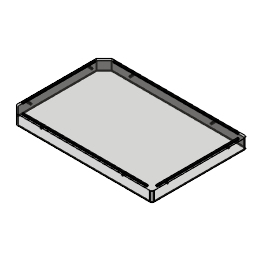
Container V3.0 (Assembly) (Autodesk Fusion 360 archive; units mm, degrees)
design "GREINER 96 WELL PLATE LID"
part number: 2026-02-05-10-27-23-618
Autodesk Fusion 360 part; units mm, degrees
(part 1 of 2)
sketch "Sketch1" plane through (0, 0, 0) normal (0, 0, 1) x (1, 0, 0)
  line L0 (61.42, -42.3) -> (-56.55, -42.3)
  line L1 (-63.55, -35.3) -> (-63.55, 35.3)
  line L2 (-56.55, 42.3) -> (61.42, 42.3)
  line L3 (63.55, 40.17) -> (63.55, -40.17)
  line L4 (63.55, -42.3) -> (-63.55, 42.3) construction
  line L5 (-63.55, -42.3) -> (63.55, 42.3) construction
  line L6 (-56.55, 42.3) -> (-63.55, 35.3)
  line L7 (0, -42.3) -> (0, 42.3) construction
  line L8 (63.55, 0) -> (-63.55, 0) construction
  line L9 (-56.55, -42.3) -> (-63.55, -35.3)
  arc A0 (63.55, 40.17) -> (61.42, 42.3) centre (61.42, 40.17) ccw
  arc A1 (61.42, -42.3) -> (63.55, -40.17) centre (61.42, -40.17) ccw
  dimension "d1" = 84.6
  dimension "d2" = 127.1
  dimension "d3" = 7
  dimension "d4" = 7
  dimension "d5" = 2.13
  constraint horizontal L0
  constraint perpendicular L0 L1
  constraint parallel L0 L2
  constraint parallel L1 L3
  constraint coincident L4 origin
  constraint coincident L5 origin
  constraint coincident L4.end L2
  constraint coincident L4.end L1
  constraint coincident L2 L7.end
  constraint perpendicular L2 L7
  constraint coincident L1 L8.end
  constraint perpendicular L1 L8
  constraint symmetric L2.start L8 L0.end
  constraint symmetric L1.end L8 L1.start
  constraint coincident L0 L7.start
  constraint coincident L3 L8.start
  constraint coincident L5.end L2
  constraint coincident L5.end L3
  constraint tangent L2 A0
  constraint tangent L3 A0
  constraint symmetric L8 L2.end L0.start
  constraint symmetric L8 L3.start L3.end
  constraint symmetric L8 A0 A1
  measures "d1" distance of L5.start L4.end
  measures "d2" distance of L4.end L5.end
  measures "d3" distance of L4.end L2.start
  measures "d4" distance of L4.end L1.end
  measures "d5" radius of A0
extrude "Extrude1" add sketch "Sketch1" against normal blind 9
sketch "Sketch2" plane through (0, 0, -9) normal (0, 0, -1) x (1, 0, 0)
  line L0 (61.42, 42.3) -> (-56.55, 42.3)
  line L1 (-56.55, 42.3) -> (-63.55, 35.3)
  line L2 (-63.55, 35.3) -> (-63.55, -35.3)
  line L3 (-63.55, -35.3) -> (-56.55, -42.3)
  line L4 (-56.55, -42.3) -> (61.42, -42.3)
  arc A0 (61.42, -42.3) -> (63.55, -40.17) centre (61.42, -40.17) ccw
  line L5 (63.55, -40.17) -> (63.55, 40.17)
  arc A1 (63.55, 40.17) -> (61.42, 42.3) centre (61.42, 40.17) ccw
  line L6 (61.42, -41.3) -> (-56.1358, -41.3)
  line L7 (-62.55, -34.8858) -> (-62.55, 34.8858)
  line L8 (-56.1358, 41.3) -> (61.42, 41.3)
  line L9 (62.55, 40.17) -> (62.55, -40.17)
  line L10 (62.55, -41.3) -> (-62.55, 41.3) construction
  line L11 (-62.55, -41.3) -> (62.55, 41.3) construction
  line L12 (-56.1358, 41.3) -> (-62.55, 34.8858)
  arc A2 (62.55, 40.17) -> (61.42, 41.3) centre (61.42, 40.17) ccw
  line L13 (63.55, 0) -> (-63.55, 0) construction
  line L14 (-56.1358, -41.3) -> (-62.55, -34.8858)
  arc A3 (61.42, -41.3) -> (62.55, -40.17) centre (61.42, -40.17) ccw
  dimension "d8" = 125.1
  dimension "d9" = 82.6
  dimension "d10" = 6.4142
  dimension "d11" = 6.4142
  dimension "d12" = 1
  dimension "d13" = 1.13
  constraint horizontal L6
  constraint perpendicular L6 L7
  constraint parallel L6 L8
  constraint parallel L7 L9
  constraint coincident L10 origin
  constraint coincident L11 origin
  constraint coincident L10.end L8
  constraint coincident L10.end L7
  constraint coincident L11.end L9
  constraint coincident L11.end L8
  constraint tangent L9 A2
  constraint tangent L8 A2
  constraint midpoint L5 L13.start
  constraint midpoint L2 L13.end
  constraint symmetric L8.start L13 L6.end
  constraint symmetric L7.end L13 L7.start
  constraint symmetric L9.start L13 L9.end
  constraint symmetric L8.end L13 L6.start
  constraint symmetric A2 L13 A3
  measures "d8" distance of L10.end L11.end
  measures "d9" distance of L11.start L10.end
  measures "d10" distance of L10.end L8.start
  measures "d11" distance of L10.end L7.end
  measures "d12" distance of L1 L12
  measures "d13" radius of A2
extrude "Extrude2" cut sketch "Sketch2" against normal blind 8 contours L6 L7 L8 L9 L12 A2 L14 A3
sketch "Sketch3" plane through (0, 0, -1) normal (0, 0, -1) x (1, 0, 0)
  line L0 (-56.1358, -41.3) -> (61.42, -41.3)
  arc A0 (61.42, -41.3) -> (62.55, -40.17) centre (61.42, -40.17) ccw
  line L1 (62.55, -40.17) -> (62.55, 40.17)
  arc A1 (62.55, 40.17) -> (61.42, 41.3) centre (61.42, 40.17) ccw
  line L2 (61.42, 41.3) -> (-56.1358, 41.3)
  line L3 (-56.1358, 41.3) -> (-62.55, 34.8858)
  line L4 (-62.55, 34.8858) -> (-62.55, -34.8858)
  line L5 (-62.55, -34.8858) -> (-56.1358, -41.3)
  line L6 (-62.55, 32.8642) -> (-35.55, 32.8642) construction
  line L7 (-35.55, 32.8642) -> (-35.55, 41.3) construction
  line L8 (-35.55, 41.3) -> (-36.55, 41.3)
  line L9 (-36.55, 41.3) -> (-36.55, 37.5)
  line L10 (-36.55, 37.5) -> (-35.55, 37.5)
  line L11 (-35.55, 37.5) -> (-35.55, 41.3)
  line L12 (-50.2731, 41.3) -> (-50.2731, 26.6) construction
  line L13 (-50.2731, 26.6) -> (-62.55, 26.6) construction
  line L14 (-62.55, 26.6) -> (-58.75, 26.6)
  line L15 (-58.75, 26.6) -> (-58.75, 27.6)
  line L16 (-58.75, 27.6) -> (-62.55, 27.6)
  line L17 (-62.55, 27.6) -> (-62.55, 26.6)
  line L18 (62.55, 0) -> (-62.55, 0) construction
  line L19 (-62.55, 30.673) -> (-62.55, 55) construction
  line L20 (62.55, 34.8173) -> (62.55, 55) construction
  line L21 (62.55, 55) -> (-62.55, 55) construction
  line L22 (0, 55) -> (0, -41.3) construction
  line L23 (62.55, 27.6) -> (62.55, 26.6)
  line L24 (62.55, 26.6) -> (58.75, 26.6)
  line L25 (58.75, 27.6) -> (62.55, 27.6)
  line L26 (58.75, 26.6) -> (58.75, 27.6)
  line L27 (36.55, 41.3) -> (36.55, 37.5)
  line L28 (35.55, 37.5) -> (35.55, 41.3)
  line L29 (36.55, 37.5) -> (35.55, 37.5)
  line L30 (35.55, 41.3) -> (36.55, 41.3)
  line L31 (62.55, -26.6) -> (58.75, -26.6)
  line L32 (58.75, -27.6) -> (62.55, -27.6)
  line L33 (58.75, -26.6) -> (58.75, -27.6)
  line L34 (35.55, -37.5) -> (35.55, -41.3)
  line L35 (36.55, -37.5) -> (35.55, -37.5)
  line L36 (36.55, -41.3) -> (36.55, -37.5)
  line L37 (62.55, -27.6) -> (62.55, -26.6)
  line L38 (35.55, -41.3) -> (36.55, -41.3)
  line L39 (-58.75, -26.6) -> (-58.75, -27.6)
  line L40 (-62.55, -26.6) -> (-58.75, -26.6)
  line L41 (-58.75, -27.6) -> (-62.55, -27.6)
  line L42 (-62.55, -27.6) -> (-62.55, -26.6)
  line L43 (-36.55, -37.5) -> (-35.55, -37.5)
  line L44 (-35.55, -37.5) -> (-35.55, -41.3)
  line L45 (-36.55, -41.3) -> (-36.55, -37.5)
  line L46 (-35.55, -41.3) -> (-36.55, -41.3)
  dimension "d16" = 27
  dimension "d17" = 3.8
  dimension "d18" = 1
  dimension "d19" = 14.7
  dimension "d20" = 3.8
  dimension "d21" = 1
  constraint coincident L4 L6.start
  constraint perpendicular L4 L6
  constraint coincident L2 L7.end
  constraint perpendicular L2 L7
  constraint horizontal L8
  constraint vertical L9
  constraint horizontal L10
  constraint vertical L11
  constraint coincident L2 L12.start
  constraint perpendicular L2 L12
  constraint coincident L4 L13.end
  constraint perpendicular L4 L13
  constraint horizontal L14
  constraint vertical L15
  constraint horizontal L16
  constraint vertical L17
  constraint midpoint L1 L18.start
  constraint midpoint L4 L18.end
  constraint coincident L4 L19.start
  constraint perpendicular L6 L19
  constraint coincident L1 L20.start
  constraint parallel L1 L20
  constraint perpendicular L19 L21
  constraint midpoint L21 L22.start
  constraint coincident L0 L22.end
  constraint perpendicular L0 L22
  constraint symmetric L7.end L22 L28.end
  constraint symmetric L8.end L22 L27.start
  constraint symmetric L9.end L22 L27.end
  constraint symmetric L10.end L22 L28.start
  constraint symmetric L13.end L22 L23.end
  constraint symmetric L14.end L22 L24.end
  constraint symmetric L15.end L22 L25.start
  constraint symmetric L16.end L22 L23.start
  constraint symmetric L7.end L18 L44.end
  constraint symmetric L8.end L18 L45.start
  constraint symmetric L9.end L18 L43.start
  constraint symmetric L10.end L18 L43.end
  constraint symmetric L13.end L18 L40.start
  constraint symmetric L14.end L18 L39.start
  constraint symmetric L15.end L18 L39.end
  constraint symmetric L16.end L18 L41.end
  constraint symmetric L18 L23.start L32.end
  constraint symmetric L18 L23.end L31.start
  constraint symmetric L18 L27.end L35.start
  constraint symmetric L18 L28.start L34.start
  constraint symmetric L18 L24.end L31.end
  constraint symmetric L18 L25.start L32.start
  constraint symmetric L18 L27.start L36.start
  constraint symmetric L18 L28.end L34.end
  measures "d16" distance of L6.start L6.end
  measures "d17" distance of L8.end L9.end
  measures "d18" distance of L9.end L10.end
  measures "d19" distance of L12.start L12.end
  measures "d20" distance of L15.end L16.end
  measures "d21" distance of L14.end L15.end
extrude "Extrude3" add sketch "Sketch3" along normal blind 1 contours L0 L43 L44 L45 L46 | L4 L39 L40 L41 L42 | L0 L34 L35 L36 L38 | L4 L14 L15 L16 L17 | L1 L31 L32 L33 L37 | L2 L8 L9 L10 L11 | L1 L23 L24 L25 L26 | L2 L27 L28 L29 L30
sketch "Sketch4" plane through (0, 0, 0) normal (0, 0, 1) x (-1, 0, 0)
  line L0 (56.55, 42.3) -> (-61.42, 42.3)
  arc A0 (-61.42, 42.3) -> (-63.55, 40.17) centre (-61.42, 40.17) ccw
  line L1 (-63.55, 40.17) -> (-63.55, -40.17)
  arc A1 (-63.55, -40.17) -> (-61.42, -42.3) centre (-61.42, -40.17) ccw
  line L2 (-61.42, -42.3) -> (56.55, -42.3)
  line L3 (56.55, -42.3) -> (63.55, -35.3)
  line L4 (63.55, -35.3) -> (63.55, 35.3)
  line L5 (63.55, 35.3) -> (56.55, 42.3)
  line L6 (-63.55, -34.3916) -> (-62.25, -34.3916) construction
  line L7 (-62.25, -34.3916) -> (-62.25, -36.4) construction
  line L8 (-60, -42.3) -> (-66.2, -42.3) construction
  line L9 (-63.55, -39.2433) -> (-63.55, -43.1) construction
  line L10 (-62.25, -36.4) -> (-60.95, -36.4)
  line L11 (-60.95, -36.4) -> (-60.95, 36.4)
  line L12 (-60.95, 36.4) -> (-62.25, 36.4)
  line L13 (-62.25, 36.4) -> (-62.25, -36.4)
  line L14 (-52.6219, -42.3) -> (-52.6219, -41) construction
  line L15 (-52.6219, -41) -> (-57.65, -41) construction
  line L16 (-57.65, -41) -> (53.05, -41)
  line L17 (53.05, -41) -> (53.05, -39.7)
  line L18 (53.05, -39.7) -> (-57.65, -39.7)
  line L19 (-57.65, -39.7) -> (-57.65, -41)
  line L20 (53.05, 39.7) -> (-57.65, 39.7)
  line L21 (-57.65, 41) -> (53.05, 41)
  line L22 (-57.65, 39.7) -> (-57.65, 41)
  line L23 (53.05, 41) -> (53.05, 39.7)
  line L24 (60.95, 0) -> (60.95, -32.3)
  line L25 (60.95, -32.3) -> (62.25, -32.3)
  line L26 (62.25, -32.3) -> (62.25, 0)
  line L27 (60.95, 0) -> (60.95, 32.3)
  line L28 (62.25, 32.3) -> (62.25, 0)
  line L29 (60.95, 32.3) -> (62.25, 32.3)
  line L30 (-63.55, 0) -> (60.95, 0) construction
  line L31 (62.25, 0) -> (63.55, 0) construction
  dimension "d24" = 1.3
  dimension "d25" = 5.9
  dimension "d26" = 72.8
  dimension "d27" = 1.3
  dimension "d28" = 1.3
  dimension "d29" = 5.9
  dimension "d30" = 1.3
  dimension "d31" = 110.7
  dimension "d32" = 32.3
  dimension "d33" = 1.3
  dimension "d34" = 1.3
  constraint coincident L1 L6.start
  constraint perpendicular L1 L6
  constraint perpendicular L6 L7
  constraint coincident L2 L8.start
  constraint parallel L2 L8
  constraint coincident L1 L9.start
  constraint perpendicular L2 L9
  constraint horizontal L10
  constraint vertical L11
  constraint horizontal L12
  constraint vertical L13
  constraint coincident L2 L14.start
  constraint perpendicular L2 L14
  constraint perpendicular L14 L15
  constraint horizontal L16
  constraint vertical L17
  constraint horizontal L18
  constraint vertical L19
  constraint midpoint L1 L30.start
  constraint midpoint L4 L31.end
  constraint symmetric L15.end L21.start L30
  constraint symmetric L16.end L21.end L30
  constraint symmetric L17.end L20.start L30
  constraint symmetric L18.end L20.end L30
  constraint vertical L24
  constraint horizontal L25
  constraint vertical L26
  constraint symmetric L24.end L27.end L30
  constraint symmetric L25.end L28.start L31
  constraint collinear L30 L31
  measures "d24" distance of L6.start L6.end
  measures "d25" distance of L7.end L8
  measures "d26" distance of L10.end L11.end
  measures "d27" distance of L7.end L10.end
  measures "d28" distance of L14.start L14.end
  measures "d29" distance of L9 L15.end
  measures "d30" distance of L15.end L18.end
  measures "d31" distance of L17.end L18.end
  measures "d32" distance of L24.start L24.end
  measures "d33" distance of L24.end L25.end
  measures "d34" distance of L4 L26
extrude "Extrude4" add sketch "Sketch4" along normal blind 1 contours L10 L11 L12 L13 | L16 L17 L18 L19 | L20 L21 L22 L23 | L24 L25 L26 L27 L28 L29
equation "d4 = d3"
equation "d11 = d10"

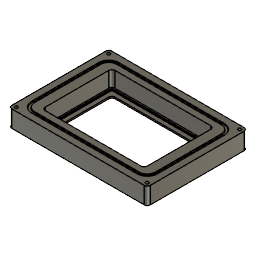
design "Base V3.0"
part number: 2026-01-30-14-30-51-369
Autodesk Fusion 360 part; units mm, degrees
sketch "Sketch1" plane through (0, 0, 0) normal (0, 0, 1) x (1, 0, 0)
  line L0 (86, -65) -> (-86, -65)
  line L1 (-90, -61) -> (-90, 61)
  line L2 (-86, 65) -> (86, 65)
  line L3 (90, 61) -> (90, -61)
  line L4 (90, -65) -> (-90, 65) construction
  line L5 (-90, -65) -> (90, 65) construction
  arc A0 (-86, 65) -> (-90, 61) centre (-86, 61) ccw
  arc A1 (90, 61) -> (86, 65) centre (86, 61) ccw
  arc A2 (86, -65) -> (90, -61) centre (86, -61) ccw
  arc A3 (-90, -61) -> (-86, -65) centre (-86, -61) ccw
  circle A4 centre (-85, 60) radius 2
  line L6 (0, 65) -> (0, -65) construction
  line L7 (90, 0) -> (-90, 0) construction
  circle A5 centre (85, 60) radius 2
  circle A6 centre (85, -60) radius 2
  circle A7 centre (-85, -60) radius 2
  dimension "d1" = 180
  dimension "d2" = 130
  dimension "d26" = 4
  dimension "d27" = 4
  dimension "d28" = 4
  dimension "d29" = 4
  dimension "d30" = 4
  dimension "d31" = 5
  dimension "d32" = 5
  constraint horizontal L0
  constraint perpendicular L0 L1
  constraint parallel L0 L2
  constraint parallel L1 L3
  constraint coincident L4 origin
  constraint coincident L5 origin
  constraint coincident L4.end L2
  constraint coincident L4.end L1
  constraint tangent L2 A0
  constraint tangent L1 A0
  constraint coincident L5.end L3
  constraint coincident L5.end L2
  constraint tangent L3 A1
  constraint tangent L2 A1
  constraint coincident L4.start L3
  constraint coincident L4.start L0
  constraint tangent L3 A2
  constraint tangent L0 A2
  constraint coincident L5.start L1
  constraint coincident L5.start L0
  constraint tangent L1 A3
  constraint tangent L0 A3
  constraint midpoint L2 L6.start
  constraint midpoint L0 L6.end
  constraint midpoint L3 L7.start
  constraint midpoint L1 L7.end
  constraint symmetric A4 L6 A5
  constraint symmetric A4 L7 A7
  constraint symmetric L7 A5 A6
  measures "d1" distance of L4.end L5.end
  measures "d2" distance of L5.start L4.end
  measures "d26" radius of A0
  measures "d27" radius of A1
  measures "d28" radius of A2
  measures "d29" radius of A3
  measures "d30" diameter of A4
  measures "d31" distance of L2 A4.centre
  measures "d32" distance of L1 A4.centre
extrude "Extrude1" add sketch "Sketch1" along normal blind 22
sketch "Sketch2" plane through (0, 0, 22) normal (0, 0, 1) x (-1, 0, 0)
  line L0 (-86, -65) -> (86, -65)
  line L1 (90, -61) -> (90, 61)
  line L2 (86, 65) -> (-86, 65)
  line L3 (-90, 61) -> (-90, -61)
  line L4 (-62.2, 45.25) -> (62.2, 45.25)
  line L5 (66.2, 41.25) -> (66.2, -41.25)
  line L6 (62.2, -45.25) -> (-62.2, -45.25)
  line L7 (-66.2, -41.25) -> (-66.2, 41.25)
  line L8 (-66.2, 45.25) -> (66.2, -45.25) construction
  line L9 (66.2, 45.25) -> (-66.2, -45.25) construction
  arc A0 (86, -65) -> (90, -61) centre (86, -61) ccw
  arc A1 (90, 61) -> (86, 65) centre (86, 61) ccw
  arc A2 (-86, 65) -> (-90, 61) centre (-86, 61) ccw
  arc A3 (-90, -61) -> (-86, -65) centre (-86, -61) ccw
  circle A4 centre (85, 60) radius 2
  circle A5 centre (-85, 60) radius 2
  circle A6 centre (-85, -60) radius 2
  circle A7 centre (85, -60) radius 2
  arc A8 (62.2, -45.25) -> (66.2, -41.25) centre (62.2, -41.25) ccw
  arc A9 (-66.2, -41.25) -> (-62.2, -45.25) centre (-62.2, -41.25) ccw
  arc A10 (66.2, 41.25) -> (62.2, 45.25) centre (62.2, 41.25) ccw
  arc A11 (-62.2, 45.25) -> (-66.2, 41.25) centre (-62.2, 41.25) ccw
  dimension "d5" = 132.4
  dimension "d6" = 90.5
  dimension "d52" = 4
  dimension "d53" = 4
  dimension "d54" = 4
  dimension "d55" = 4
  constraint horizontal L4
  constraint perpendicular L4 L5
  constraint parallel L4 L6
  constraint parallel L5 L7
  constraint coincident L8 origin
  constraint coincident L9 origin
  constraint coincident L8.end L6
  constraint coincident L8.end L5
  constraint tangent L6 A8
  constraint tangent L5 A8
  constraint coincident L9.end L6
  constraint coincident L9.end L7
  constraint tangent L6 A9
  constraint tangent L7 A9
  constraint coincident L9.start L5
  constraint coincident L9.start L4
  constraint tangent L5 A10
  constraint tangent L4 A10
  constraint coincident L8.start L7
  constraint coincident L8.start L4
  constraint tangent L7 A11
  constraint tangent L4 A11
  measures "d5" distance of L8.end L9.end
  measures "d6" distance of L9.start L8.end
  measures "d52" radius of A8
  measures "d53" radius of A9
  measures "d54" radius of A10
  measures "d55" radius of A11
extrude "Extrude2" cut sketch "Sketch2" against normal blind 20 contours L4 L5 L6 L7 A8 A9 A10 A11
sketch "Sketch3" plane through (0, 0, 22) normal (0, 0, 1) x (-1, 0, 0)
  line L0 (66.2, 41.25) -> (66.2, -41.25)
  line L1 (62.2, -45.25) -> (-62.2, -45.25)
  line L2 (-66.2, -41.25) -> (-66.2, 41.25)
  line L3 (-62.2, 45.25) -> (62.2, 45.25)
  line L4 (-86, -65) -> (86, -65)
  line L5 (90, -61) -> (90, 61)
  line L6 (86, 65) -> (-86, 65)
  line L7 (-90, 61) -> (-90, -61)
  line L8 (-79.9494, 54.9494) -> (79.9494, 54.9494) construction
  line L9 (79.9494, 54.9494) -> (79.9494, -54.9494) construction
  line L10 (79.9494, -54.9494) -> (-79.9494, -54.9494) construction
  line L11 (-79.9494, -54.9494) -> (-79.9494, 54.9494) construction
  line L12 (-79.9494, 54.9494) -> (79.9494, -54.9494) construction
  line L13 (79.9494, 54.9494) -> (-79.9494, -54.9494) construction
  line L14 (78.5149, 43.2459) -> (78.5149, -43.2459)
  line L15 (68.2459, -53.5149) -> (-68.2459, -53.5149)
  line L16 (-78.5149, -43.2459) -> (-78.5149, 43.2459)
  line L17 (-69.5341, 47.3937) -> (78.5149, -53.5149) construction
  line L18 (70.6619, 45.6619) -> (-70.6619, -45.6619) construction
  line L19 (-68.2459, 56.3839) -> (68.2459, 56.3839)
  line L20 (81.3839, 43.2459) -> (81.3839, -43.2459)
  line L21 (68.2459, -56.3839) -> (-68.2459, -56.3839)
  line L22 (-81.3839, -43.2459) -> (-81.3839, 43.2459)
  line L23 (-72.429, 50.1798) -> (81.3839, -56.3839) construction
  line L24 (73.5309, 48.5309) -> (-73.5309, -48.5309) construction
  arc A0 (68.2459, -53.5149) -> (78.5149, -43.2459) centre (68.2459, -43.2459) ccw
  arc A1 (68.2459, -56.3839) -> (81.3839, -43.2459) centre (68.2459, -43.2459) ccw
  line L25 (0, -65) -> (0, 65) construction
  line L26 (-90, 0) -> (90, 0) construction
  arc A2 (-78.5149, -43.2459) -> (-68.2459, -53.5149) centre (-68.2459, -43.2459) ccw
  arc A3 (-81.3839, -43.2459) -> (-68.2459, -56.3839) centre (-68.2459, -43.2459) ccw
  arc A4 (-68.2459, 53.5149) -> (-78.5149, 43.2459) centre (-68.2459, 43.2459) ccw
  arc A5 (-68.2459, 56.3839) -> (-81.3839, 43.2459) centre (-68.2459, 43.2459) ccw
  arc A6 (78.5149, 43.2459) -> (68.2459, 53.5149) centre (68.2459, 43.2459) ccw
  arc A7 (81.3839, 43.2459) -> (68.2459, 56.3839) centre (68.2459, 43.2459) ccw
  line L27 (-68.2459, 53.5149) -> (68.2459, 53.5149)
  arc A8 (86, -65) -> (90, -61) centre (86, -61) ccw
  arc A9 (90, 61) -> (86, 65) centre (86, 61) ccw
  arc A10 (-86, 65) -> (-90, 61) centre (-86, 61) ccw
  arc A11 (-90, -61) -> (-86, -65) centre (-86, -61) ccw
  circle A12 centre (85, 60) radius 2
  circle A13 centre (-85, 60) radius 2
  circle A14 centre (-85, -60) radius 2
  circle A15 centre (85, -60) radius 2
  arc A16 (66.2, 41.25) -> (62.2, 45.25) centre (62.2, 41.25) ccw
  arc A17 (62.2, -45.25) -> (66.2, -41.25) centre (62.2, -41.25) ccw
  arc A18 (-66.2, -41.25) -> (-62.2, -45.25) centre (-62.2, -41.25) ccw
  arc A19 (-62.2, 45.25) -> (-66.2, 41.25) centre (-62.2, 41.25) ccw
  dimension "d9" = 159.8988
  dimension "d15" = 109.8988
  dimension "d16" = 1.4345
  dimension "d17" = 1.4345
  dimension "d18" = 1.4345
  dimension "d19" = 1.4345
  dimension "d20" = 10.269
  dimension "d21" = 13.138
  constraint horizontal L8
  constraint perpendicular L8 L9
  constraint parallel L8 L10
  constraint parallel L9 L11
  constraint coincident L12 origin
  constraint coincident L13 origin
  constraint parallel L15 L27
  constraint parallel L14 L16
  constraint coincident L17 origin
  constraint coincident L18 origin
  constraint horizontal L19
  constraint perpendicular L19 L20
  constraint parallel L19 L21
  constraint parallel L20 L22
  constraint coincident L23 origin
  constraint coincident L24 origin
  constraint coincident L17.end L15
  constraint coincident L17.end L14
  constraint tangent L15 A0
  constraint tangent L14 A0
  constraint coincident L23.end L21
  constraint coincident L23.end L20
  constraint tangent L21 A1
  constraint tangent L20 A1
  constraint midpoint L4 L25.start
  constraint midpoint L6 L25.end
  constraint midpoint L7 L26.start
  constraint midpoint L5 L26.end
  constraint symmetric L15.start L25 L15.end
  constraint symmetric L14.end L25 L16.start
  constraint symmetric A0 L25 A2
  constraint symmetric L21.start L25 L21.end
  constraint symmetric L20.end L25 L22.start
  constraint symmetric A1 L25 A3
  constraint symmetric L15.start L26 A6.end
  constraint symmetric L14.end L26 L14.start
  constraint symmetric A0 L26 A6
  constraint symmetric L21.start L26 L19.end
  constraint symmetric L20.end L26 L20.start
  constraint symmetric A1 L26 A7
  constraint symmetric L26 L15.end A4.start
  constraint symmetric L26 L16.start L16.end
  constraint symmetric L26 A2 A4
  constraint symmetric L26 L21.end L19.start
  constraint symmetric L26 L22.start L22.end
  constraint symmetric L26 A3 A5
  measures "d9" distance of L8.start L8.end
  measures "d15" distance of L8 L10
  measures "d16" distance of L11 L16
  measures "d17" distance of L10 L15
  measures "d18" distance of L11 L22
  measures "d19" distance of L10 L21
  measures "d20" radius of A0
  measures "d21" radius of A1
extrude "Extrude3" cut sketch "Sketch3" against normal blind 1.424 contours L19 L20 L21 L22 A1 A3 A5 A7
draft "Draft1" angle 10 neutral plane through (0, 0, 20.576) pull (0, 0, 1) 16 faces at (-78.5149, -14.4153, 21.5253) (-70.6669, 53.2254, 21.0507) (-22.7486, 53.5149, 21.5253) (74.2025, 51.6108, 21.0507) (78.5149, 14.4153, 21.0507) (71.6046, -52.9501, 21.5253) (22.7486, -53.5149, 21.5253) (-70.6669, -53.2254, 21.0507) (-81.3839, -14.4153, 21.5253) (-68.871, -56.369, 21.0507) (22.7486, -56.3839, 21.0507) (77.7543, -52.3122, 21.0507) (81.3839, 14.4153, 21.5253) (77.3122, 52.7543, 21.0507) (-22.7486, 56.3839, 21.0507) (-73.1288, 55.4428, 21.0507)
sketch "Sketch4" plane through (0, 0, 2) normal (0, 0, 1) x (-1, 0, 0)
  line L0 (-62.2, -45.25) -> (62.2, -45.25)
  line L1 (66.2, -41.25) -> (66.2, 41.25)
  line L2 (62.2, 45.25) -> (-62.2, 45.25)
  line L3 (-66.2, 41.25) -> (-66.2, -41.25)
  line L4 (-52.2, 35.25) -> (52.2, 35.25)
  line L5 (56.2, 31.25) -> (56.2, -31.25)
  line L6 (52.2, -35.25) -> (-52.2, -35.25)
  line L7 (-56.2, -31.25) -> (-56.2, 31.25)
  line L8 (-56.2, 35.25) -> (56.2, -35.25) construction
  line L9 (56.2, 35.25) -> (-56.2, -35.25) construction
  arc A0 (66.2, 41.25) -> (62.2, 45.25) centre (62.2, 41.25) ccw
  arc A1 (-62.2, 45.25) -> (-66.2, 41.25) centre (-62.2, 41.25) ccw
  arc A2 (-66.2, -41.25) -> (-62.2, -45.25) centre (-62.2, -41.25) ccw
  arc A3 (62.2, -45.25) -> (66.2, -41.25) centre (62.2, -41.25) ccw
  arc A4 (52.2, -35.25) -> (56.2, -31.25) centre (52.2, -31.25) ccw
  arc A5 (-56.2, -31.25) -> (-52.2, -35.25) centre (-52.2, -31.25) ccw
  arc A6 (-52.2, 35.25) -> (-56.2, 31.25) centre (-52.2, 31.25) ccw
  arc A7 (56.2, 31.25) -> (52.2, 35.25) centre (52.2, 31.25) ccw
  dimension "d35" = 10
  dimension "d36" = 10
  dimension "d71" = 4
  dimension "d72" = 4
  dimension "d73" = 4
  dimension "d74" = 4
  constraint horizontal L4
  constraint perpendicular L4 L5
  constraint parallel L4 L6
  constraint parallel L5 L7
  constraint coincident L8 origin
  constraint coincident L9 origin
  constraint coincident L8.end L6
  constraint coincident L8.end L5
  constraint tangent L6 A4
  constraint tangent L5 A4
  constraint coincident L9.end L6
  constraint coincident L9.end L7
  constraint tangent L6 A5
  constraint tangent L7 A5
  constraint coincident L8.start L7
  constraint coincident L8.start L4
  constraint tangent L7 A6
  constraint tangent L4 A6
  constraint coincident L9.start L4
  constraint coincident L9.start L5
  constraint tangent L4 A7
  constraint tangent L5 A7
  measures "d35" distance of L3 L7
  measures "d36" distance of L0 L6
  measures "d71" radius of A4
  measures "d72" radius of A5
  measures "d73" radius of A6
  measures "d74" radius of A7
extrude "Extrude4" cut sketch "Sketch4" against normal blind 5 contours L4 L5 L6 L7 A4 A5 A6 A7
sketch "Sketch6" plane through (0, 0, 2) normal (0, 0, 1) x (-1, 0, 0)
  line L0 (56.2, 31.25) -> (56.2, -31.25)
  line L1 (52.2, -35.25) -> (-52.2, -35.25)
  line L2 (-56.2, -31.25) -> (-56.2, 31.25)
  line L3 (-52.2, 35.25) -> (52.2, 35.25)
  arc A0 (66.2, 41.25) -> (62.2, 45.25) centre (62.2, 41.25) ccw
  line L4 (62.2, 45.25) -> (-62.2, 45.25)
  arc A1 (-62.2, 45.25) -> (-66.2, 41.25) centre (-62.2, 41.25) ccw
  line L5 (-66.2, 41.25) -> (-66.2, -41.25)
  arc A2 (-66.2, -41.25) -> (-62.2, -45.25) centre (-62.2, -41.25) ccw
  line L6 (-62.2, -45.25) -> (62.2, -45.25)
  arc A3 (62.2, -45.25) -> (66.2, -41.25) centre (62.2, -41.25) ccw
  line L7 (66.2, -41.25) -> (66.2, 41.25)
  arc A4 (60.9079, -41.3399) -> (62.4799, -39.7679) centre (60.9079, -39.7679) ccw construction
  arc A5 (-62.4799, -39.7399) -> (-60.9079, -41.3119) centre (-60.9079, -39.7399) ccw construction
  line L8 (-48.9575, -41.8399) -> (48.9575, -41.8399) construction
  line L9 (48.9575, 41.8399) -> (-48.9575, 41.8399) construction
  line L10 (-62.9799, 29.7119) -> (-62.9799, 27.8175) construction
  line L11 (48.9575, -41.8399) -> (50.8519, -41.8399) construction
  line L12 (62.4799, 30.3078) -> (62.4799, 39.7679) construction
  arc A6 (-60.88, 42.74) -> (-63.88, 39.74) centre (-60.88, 39.74) ccw construction
  line L13 (63.88, 39.74) -> (63.88, -39.74) construction
  arc A7 (63.88, 39.74) -> (60.88, 42.74) centre (60.88, 39.74) ccw construction
  line L14 (-62.9799, -29.7119) -> (-62.4799, -30.3078) construction
  line L15 (51.4478, 41.3399) -> (50.8519, 41.8399) construction
  arc A8 (60.88, -42.74) -> (63.88, -39.74) centre (60.88, -39.74) ccw construction
  line L16 (-48.9575, 41.8399) -> (-50.8519, 41.8399) construction
  line L17 (-60.88, 42.74) -> (60.88, 42.74) construction
  line L18 (-62.9799, -27.8175) -> (-62.9799, -29.7119) construction
  line L19 (60.88, -42.74) -> (-60.88, -42.74) construction
  line L20 (62.9799, 29.7119) -> (62.4799, 30.3078) construction
  line L21 (-50.8519, 41.8399) -> (-51.4811, 41.3119) construction
  line L22 (62.4799, -39.7679) -> (62.4799, -30.3078) construction
  line L23 (-50.8519, -41.8399) -> (-48.9575, -41.8399) construction
  line L24 (60.9079, 41.3399) -> (51.4478, 41.3399) construction
  line L25 (50.8519, 41.8399) -> (48.9575, 41.8399) construction
  line L26 (62.9799, 27.8175) -> (62.9799, 29.7119) construction
  line L27 (51.4478, -41.3399) -> (60.9079, -41.3399) construction
  line L28 (62.9799, -27.8175) -> (62.9799, 27.8175) construction
  line L29 (-63.88, -39.74) -> (-63.88, 39.74) construction
  line L30 (50.8519, -41.8399) -> (51.4478, -41.3399) construction
  line L31 (62.9799, -29.7119) -> (62.9799, -27.8175) construction
  arc A9 (-63.88, -39.74) -> (-60.88, -42.74) centre (-60.88, -39.74) ccw construction
  arc A10 (62.4799, 39.7679) -> (60.9079, 41.3399) centre (60.9079, 39.7679) ccw construction
  line L32 (62.4799, -30.3078) -> (62.9799, -29.7119) construction
  line L33 (-62.4799, 30.3078) -> (-62.9799, 29.7119) construction
  line L34 (-60.9079, -41.3119) -> (-51.4811, -41.3119) construction
  arc A11 (-60.9079, 41.3119) -> (-62.4799, 39.7399) centre (-60.9079, 39.7399) ccw construction
  line L35 (-51.4811, -41.3119) -> (-50.8519, -41.8399) construction
  line L36 (-51.4811, 41.3119) -> (-60.9079, 41.3119) construction
  line L37 (-62.4799, 39.7399) -> (-62.4799, 30.3078) construction
  line L38 (-62.4799, -30.3078) -> (-62.4799, -39.7399) construction
  line L39 (-62.9799, 27.8175) -> (-62.9799, -27.8175) construction
  line L40 (0, -45.25) -> (0, 45.25) construction
  line L41 (-66.2, 0) -> (66.2, 0) construction
  line L42 (-60.85, 43.25) -> (60.85, 43.25)
  line L43 (64.35, 39.75) -> (64.35, -39.75)
  line L44 (60.85, -43.25) -> (-60.85, -43.25)
  line L45 (-64.35, -39.75) -> (-64.35, 39.75)
  line L46 (-64.35, 43.25) -> (64.35, -43.25) construction
  line L47 (64.35, 43.25) -> (-64.35, -43.25) construction
  arc A12 (60.85, -43.25) -> (64.35, -39.75) centre (60.85, -39.75) ccw
  arc A13 (-64.35, -39.75) -> (-60.85, -43.25) centre (-60.85, -39.75) ccw
  arc A14 (-60.85, 43.25) -> (-64.35, 39.75) centre (-60.85, 39.75) ccw
  arc A15 (64.35, 39.75) -> (60.85, 43.25) centre (60.85, 39.75) ccw
  line L48 (-60.85, 40.75) -> (60.85, 40.75)
  line L49 (61.85, 39.75) -> (61.85, -39.75)
  line L50 (60.85, -40.75) -> (-60.85, -40.75)
  line L51 (-61.85, -39.75) -> (-61.85, 39.75)
  line L52 (-61.85, 40.75) -> (61.85, -40.75) construction
  line L53 (61.85, 40.75) -> (-61.85, -40.75) construction
  arc A16 (-61.85, -39.75) -> (-60.85, -40.75) centre (-60.85, -39.75) ccw
  arc A17 (60.85, -40.75) -> (61.85, -39.75) centre (60.85, -39.75) ccw
  arc A18 (61.85, 39.75) -> (60.85, 40.75) centre (60.85, 39.75) ccw
  arc A19 (-60.85, 40.75) -> (-61.85, 39.75) centre (-60.85, 39.75) ccw
  arc A20 (52.2, -35.25) -> (56.2, -31.25) centre (52.2, -31.25) ccw
  arc A21 (-56.2, -31.25) -> (-52.2, -35.25) centre (-52.2, -31.25) ccw
  arc A22 (-52.2, 35.25) -> (-56.2, 31.25) centre (-52.2, 31.25) ccw
  arc A23 (56.2, 31.25) -> (52.2, 35.25) centre (52.2, 31.25) ccw
  dimension "d56" = 128.7
  dimension "d57" = 86.5
  dimension "d58" = 3.5
  dimension "d59" = 3.5
  dimension "d60" = 3.5
  dimension "d61" = 3.5
  dimension "d63" = 2.5
  dimension "d64" = 2.5
  dimension "d65" = 1
  dimension "d66" = 1
  dimension "d67" = 1
  dimension "d68" = 1
  constraint midpoint L6 L40.start
  constraint midpoint L4 L40.end
  constraint midpoint L5 L41.start
  constraint midpoint L7 L41.end
  constraint horizontal L42
  constraint perpendicular L42 L43
  constraint parallel L42 L44
  constraint parallel L43 L45
  constraint coincident L46 origin
  constraint coincident L47 origin
  constraint coincident L46.end L44
  constraint coincident L46.end L43
  constraint tangent L44 A12
  constraint tangent L43 A12
  constraint coincident L47.end L45
  constraint coincident L47.end L44
  constraint tangent L45 A13
  constraint tangent L44 A13
  constraint coincident L46.start L45
  constraint coincident L46.start L42
  constraint tangent L45 A14
  constraint tangent L42 A14
  constraint coincident L47.start L42
  constraint coincident L47.start L43
  constraint tangent L42 A15
  constraint tangent L43 A15
  constraint horizontal L48
  constraint perpendicular L48 L49
  constraint parallel L48 L50
  constraint parallel L49 L51
  constraint coincident L52 origin
  constraint coincident L53 origin
  constraint coincident L53.end L51
  constraint coincident L53.end L50
  constraint tangent L51 A16
  constraint tangent L50 A16
  constraint coincident L52.end L50
  constraint coincident L52.end L49
  constraint tangent L50 A17
  constraint tangent L49 A17
  constraint coincident L53.start L48
  constraint coincident L53.start L49
  constraint tangent L48 A18
  constraint tangent L49 A18
  constraint coincident L52.start L51
  constraint coincident L52.start L48
  constraint tangent L51 A19
  constraint tangent L48 A19
  measures "d56" distance of L46.end L47.end
  measures "d57" distance of L47.start L46.end
  measures "d58" radius of A12
  measures "d59" radius of A13
  measures "d60" radius of A14
  measures "d61" radius of A15
  measures "d63" distance of L45 L51
  measures "d64" distance of L44 L50
  measures "d65" radius of A16
  measures "d66" radius of A17
  measures "d67" radius of A18
  measures "d68" radius of A19
extrude "Extrude6" cut sketch "Sketch6" against normal blind 1 contours L42 L43 L44 L45 A12 A13 A14 A15
equation "d9 = ( ORingPerimeter - 100 mm ) / 4 + 50 mm"
equation "ORingDiameter = 1.78 mm" comment "Diamter of the O ring"
equation "ORingInnerDiameter = 170 mm" comment "Inner diamter of the o ring bore"
equation "ORingPerimeter = 2 * 3.1412 * ( ( ORingInnerDiameter / 2 ) + ORingDiameter / 2 )"
equation "PanelWidth = 80 mm"
equation "PanelLength = 115 mm"
equation "d15 = ( ORingPerimeter - 100 mm ) / 4"
equation "d16 = ( ( ORingDiameter * 1.05 ) / 2 ) + 0.5 mm"
equation "d17 = ( ( ORingDiameter * 1.05 ) / 2 ) + 0.5 mm"
equation "d18 = ( ( ORingDiameter * 1.05 ) / 2 ) + 0.5 mm"
equation "d19 = ( ( ORingDiameter * 1.05 ) / 2 ) + 0.5 mm"
equation "d20 = ( ORingDiameter ) * 6 + ORingDiameter * 0.05 - 0.5 mm"
equation "d21 = ( ORingDiameter ) * 6 + ( ORingDiameter * 1.1 ) + 0.5 mm"
equation "d22 = -ORingDiameter * 0.8"
equation "ORing2Diameter = 2 mm" comment "Second O ring Diameter"
equation "ORing2InnerDiameter = 126 mm" comment "Inner diameter of the second O Ring"
equation "ORing2Perimeter = 2 * 3.1412 * ( ( ORing2InnerDiameter / 2 ) + ORing2Diameter / 2 )"

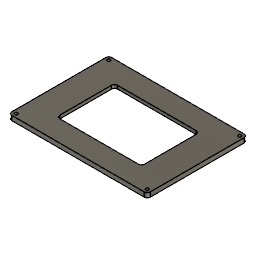
design "Lid V3.0"
part number: 2026-01-29-14-58-12-979
Autodesk Fusion 360 part; units mm, degrees
sketch "Sketch2" plane through (0, 0, 0) normal (0, 0, 1) x (1, 0, 0)
  line L0 (-46, 50) -> (126, 50)
  line L1 (130, 46) -> (130, -76)
  line L2 (126, -80) -> (-46, -80)
  line L3 (-50, -76) -> (-50, 46)
  circle A0 centre (-45, 45) radius 2
  line L4 (40, -80) -> (40, 50) construction
  line L5 (-50, -15) -> (130, -15) construction
  arc A1 (-46, 50) -> (-50, 46) centre (-46, 46) ccw
  circle A2 centre (125, 45) radius 2
  arc A3 (130, 46) -> (126, 50) centre (126, 46) ccw
  circle A4 centre (125, -75) radius 2
  arc A5 (126, -80) -> (130, -76) centre (126, -76) ccw
  circle A6 centre (-45, -75) radius 2
  arc A7 (-50, -76) -> (-46, -80) centre (-46, -76) ccw
  point P0 (-50, 50)
  point P1 (130, 50)
  dimension "d3" = 4
  dimension "d4" = 5
  dimension "d5" = 5
  dimension "d6" = 4
  dimension "d63" = 180
  dimension "d64" = 130
  constraint horizontal L0
  constraint vertical L1
  constraint horizontal L2
  constraint vertical L3
  constraint coincident L0 L4.end
  constraint coincident L3 L5.start
  constraint coincident P0 L0
  constraint coincident P0 L3
  constraint tangent L0 A1
  constraint tangent L3 A1
  constraint symmetric P0 L4 P1
  constraint symmetric A0 L4 A2
  constraint symmetric L4 L0.start L0.end
  constraint symmetric L4 L3.end L1.start
  constraint symmetric L4 A1 A3
  constraint coincident L1 L5.end
  constraint symmetric A0 L5 A6
  constraint symmetric L5 L0.start L2.end
  constraint symmetric L5 L3.end L3.start
  constraint symmetric L5 A1 A7
  constraint symmetric L5 L1.start L1.end
  constraint symmetric L5 L0.end L2.start
  constraint symmetric L5 A2 A4
  constraint symmetric L5 A3 A5
  constraint coincident L2 L4.start
  measures "d3" diameter of A0
  measures "d4" distance of L0 A0.centre
  measures "d5" distance of L3 A0.centre
  measures "d6" radius of A1
  measures "d63" distance of L1 L3
  measures "d64" distance of L0 L2
extrude "Extrude1" add sketch "Sketch2" along normal blind 6
sketch "Sketch3" plane through (0, 0, 0) normal (0, 0, -1) x (1, 0, 0)
  circle A0 centre (125, 75) radius 2
  circle A1 centre (-45, 75) radius 2
  circle A2 centre (-45, -45) radius 2
  circle A3 centre (125, -45) radius 2
  arc A4 (-50, -46) -> (-46, -50) centre (-46, -46) ccw
  line L0 (-46, -50) -> (126, -50)
  arc A5 (126, -50) -> (130, -46) centre (126, -46) ccw
  line L1 (130, -46) -> (130, 76)
  arc A6 (130, 76) -> (126, 80) centre (126, 76) ccw
  line L2 (126, 80) -> (-46, 80)
  arc A7 (-46, 80) -> (-50, 76) centre (-46, 76) ccw
  line L3 (-50, 76) -> (-50, -46)
  line L4 (40, 80) -> (40, -50) construction
  line L5 (130, 15) -> (-50, 15) construction
  line L6 (119.9494, -39.9494) -> (-39.9494, -39.9494) construction
  line L7 (-39.9494, -39.9494) -> (-39.9494, 69.9494) construction
  line L8 (-39.9494, 69.9494) -> (119.9494, 69.9494) construction
  line L9 (119.9494, 69.9494) -> (119.9494, -39.9494) construction
  line L10 (119.9494, -39.9494) -> (-39.9494, 69.9494) construction
  line L11 (-39.9494, -39.9494) -> (119.9494, 69.9494) construction
  line L12 (108.2459, -41.3839) -> (-28.2459, -41.3839)
  line L13 (-41.3839, -28.2459) -> (-41.3839, 58.2459)
  line L14 (-28.2459, 71.3839) -> (108.2459, 71.3839)
  line L15 (121.3839, 58.2459) -> (121.3839, -28.2459)
  line L16 (95.6336, -23.5438) -> (-41.3839, 71.3839) construction
  line L17 (-38.6963, -33.1786) -> (83.6146, 41.7012) construction
  line L18 (-38.5149, -28.2459) -> (-38.5149, 58.2459)
  line L19 (-28.2459, 68.5149) -> (108.2459, 68.5149)
  line L20 (118.5149, 58.2459) -> (118.5149, -28.2459)
  line L21 (104.513, -28.9713) -> (-38.5149, 68.5149) construction
  line L22 (-36.0332, -30.305) -> (80.8211, 39.3236) construction
  arc A8 (-28.2459, 68.5149) -> (-38.5149, 58.2459) centre (-28.2459, 58.2459) ccw
  arc A9 (-28.2459, 71.3839) -> (-41.3839, 58.2459) centre (-28.2459, 58.2459) ccw
  arc A10 (118.5149, 58.2459) -> (108.2459, 68.5149) centre (108.2459, 58.2459) ccw
  arc A11 (121.3839, 58.2459) -> (108.2459, 71.3839) centre (108.2459, 58.2459) ccw
  arc A12 (-38.5149, -28.2459) -> (-28.2459, -38.5149) centre (-28.2459, -28.2459) ccw
  arc A13 (-41.3839, -28.2459) -> (-28.2459, -41.3839) centre (-28.2459, -28.2459) ccw
  arc A14 (108.2459, -38.5149) -> (118.5149, -28.2459) centre (108.2459, -28.2459) ccw
  arc A15 (108.2459, -41.3839) -> (121.3839, -28.2459) centre (108.2459, -28.2459) ccw
  line L23 (108.2459, -38.5149) -> (-28.2459, -38.5149)
  point P0 (40, 15)
  point P1 (40, 15)
  point P2 (40, 15)
  point P3 (40, 15)
  point P4 (40, 15)
  dimension "d25" = 159.8988
  dimension "d27" = 109.8988
  dimension "d28" = 1.4345
  dimension "d29" = 1.4345
  dimension "d30" = 1.4345
  dimension "d31" = 1.4345
  dimension "d44" = 10.269
  dimension "d45" = 13.138
  constraint midpoint L2 L4.start
  constraint midpoint L0 L4.end
  constraint midpoint L1 L5.start
  constraint midpoint L3 L5.end
  constraint midpoint L4 P4
  constraint coincident P4 P3
  constraint horizontal L6
  constraint perpendicular L6 L7
  constraint parallel L6 L8
  constraint parallel L7 L9
  constraint coincident L10 P4
  constraint coincident L11 P4
  constraint horizontal L12
  constraint perpendicular L12 L13
  constraint parallel L12 L14
  constraint parallel L13 L15
  constraint coincident L16 P4
  constraint coincident L17 P4
  constraint perpendicular L18 L23
  constraint parallel L19 L23
  constraint parallel L18 L20
  constraint coincident L21 P4
  constraint coincident L22 P4
  constraint coincident L21.end L19
  constraint coincident L21.end L18
  constraint tangent L19 A8
  constraint tangent L18 A8
  constraint coincident L16.end L14
  constraint coincident L16.end L13
  constraint tangent L14 A9
  constraint tangent L13 A9
  constraint symmetric L4 L19.start L19.end
  constraint symmetric L4 L18.end L20.start
  constraint symmetric L4 A8 A10
  constraint symmetric L4 L14.start L14.end
  constraint symmetric L4 L13.end L15.start
  constraint symmetric L4 A9 A11
  constraint symmetric L5 L19.start A12.end
  constraint symmetric L5 L18.end L18.start
  constraint symmetric L5 A8 A12
  constraint symmetric L5 L14.start L12.end
  constraint symmetric L5 L13.end L13.start
  constraint symmetric L5 A9 A13
  constraint symmetric L5 L19.end A14.start
  constraint symmetric L5 L20.start L20.end
  constraint symmetric L5 A10 A14
  constraint symmetric L5 L14.end L12.start
  constraint symmetric L5 L15.start L15.end
  constraint symmetric L5 A11 A15
  measures "d25" distance of L7.end L8.end
  measures "d27" distance of L6.end L7.end
  measures "d28" distance of L9 L15
  measures "d29" distance of L8 L14
  measures "d30" distance of L8 L19
  measures "d31" distance of L9 L20
  measures "d44" radius of A8
  measures "d45" radius of A9
extrude "Extrude4" add sketch "Sketch3" along normal blind 1.424 contours L12 L13 L14 L15 A9 A11 A13 A15
draft "Draft3" angle 10 neutral plane through (0, 0, -1.424) pull (0, 0, -1) 16 faces at (62.7486, -68.5149, -0.9493) (117.7793, -62.0625, -0.9493) (118.5149, -29.4153, -0.4747) (115.6779, 35.3323, -0.9493) (62.7486, 38.5149, -0.4747) (-32.9514, 37.3734, -0.9493) (-38.5149, -29.4153, -0.9493) (-35.6779, -65.3323, -0.9493) (-41.3839, -0.5847, -0.4747) (-33.1288, 40.4428, -0.9493) (17.2514, 41.3839, -0.9493) (116.3673, 38.5731, -0.9493) (121.3839, -29.4153, -0.9493) (119.6238, -64.8149, -0.9493) (62.7486, -71.3839, -0.9493) (-38.9478, -65.8667, -0.9493)
sketch "Sketch5" plane through (0, 0, -1.424) normal (0, 0, -1) x (1, 0, 0)
  line L0 (-28.2459, 68.5149) -> (108.2459, 68.5149)
  line L1 (118.5149, 58.2459) -> (118.5149, -28.2459)
  line L2 (108.2459, -38.5149) -> (-28.2459, -38.5149)
  line L3 (-38.5149, -28.2459) -> (-38.5149, 58.2459)
  line L4 (108.2459, 71.3839) -> (-28.2459, 71.3839)
  line L5 (-41.3839, 58.2459) -> (-41.3839, -28.2459)
  line L6 (-28.2459, -41.3839) -> (108.2459, -41.3839)
  line L7 (121.3839, -28.2459) -> (121.3839, 58.2459)
  line L8 (40, 71.3839) -> (40, -41.3839) construction
  line L9 (121.3839, 15) -> (-41.3839, 15) construction
  line L10 (119.9494, -39.9494) -> (-39.9494, -39.9494) construction
  line L11 (-39.9494, -39.9494) -> (-39.9494, 69.9494) construction
  line L12 (-39.9494, 69.9494) -> (119.9494, 69.9494) construction
  line L13 (119.9494, 69.9494) -> (119.9494, -39.9494) construction
  line L14 (119.9494, -39.9494) -> (-39.9494, 69.9494) construction
  line L15 (-39.9494, -39.9494) -> (119.9494, 69.9494) construction
  line L16 (108.2459, -40.8839) -> (-28.2459, -40.8839)
  line L17 (-40.8839, -28.2459) -> (-40.8839, 58.2459)
  line L18 (-28.2459, 70.8839) -> (108.2459, 70.8839)
  line L19 (120.8839, 58.2459) -> (120.8839, -28.2459)
  line L20 (98.0985, -25.1411) -> (-40.8839, 70.8839) construction
  line L21 (-40.8839, -40.8839) -> (98.0985, 55.1411) construction
  line L22 (108.2459, -39.0149) -> (-28.2459, -39.0149)
  line L23 (-39.0149, -28.2459) -> (-39.0149, 58.2459)
  line L24 (119.0149, 58.2459) -> (119.0149, -28.2459)
  line L25 (97.1479, -24.0666) -> (-39.0149, 69.0149) construction
  line L26 (-39.0149, -39.0149) -> (97.1479, 54.0666) construction
  arc A0 (118.5149, 58.2459) -> (108.2459, 68.5149) centre (108.2459, 58.2459) ccw
  arc A1 (108.2459, -38.5149) -> (118.5149, -28.2459) centre (108.2459, -28.2459) ccw
  arc A2 (-38.5149, -28.2459) -> (-28.2459, -38.5149) centre (-28.2459, -28.2459) ccw
  arc A3 (-28.2459, 68.5149) -> (-38.5149, 58.2459) centre (-28.2459, 58.2459) ccw
  arc A4 (-41.3839, -28.2459) -> (-28.2459, -41.3839) centre (-28.2459, -28.2459) ccw
  arc A5 (108.2459, -41.3839) -> (121.3839, -28.2459) centre (108.2459, -28.2459) ccw
  arc A6 (121.3839, 58.2459) -> (108.2459, 71.3839) centre (108.2459, 58.2459) ccw
  arc A7 (-28.2459, 71.3839) -> (-41.3839, 58.2459) centre (-28.2459, 58.2459) ccw
  arc A8 (-28.2459, 69.0149) -> (-39.0149, 58.2459) centre (-28.2459, 58.2459) ccw
  arc A9 (-28.2459, 70.8839) -> (-40.8839, 58.2459) centre (-28.2459, 58.2459) ccw
  arc A10 (119.0149, 58.2459) -> (108.2459, 69.0149) centre (108.2459, 58.2459) ccw
  arc A11 (120.8839, 58.2459) -> (108.2459, 70.8839) centre (108.2459, 58.2459) ccw
  line L27 (-28.2459, 69.0149) -> (108.2459, 69.0149)
  arc A12 (108.2459, -39.0149) -> (119.0149, -28.2459) centre (108.2459, -28.2459) ccw
  arc A13 (108.2459, -40.8839) -> (120.8839, -28.2459) centre (108.2459, -28.2459) ccw
  arc A14 (-39.0149, -28.2459) -> (-28.2459, -39.0149) centre (-28.2459, -28.2459) ccw
  arc A15 (-40.8839, -28.2459) -> (-28.2459, -40.8839) centre (-28.2459, -28.2459) ccw
  point P0 (40, 15)
  point P1 (40, 15)
  point P2 (40, 15)
  dimension "d36" = 159.8988
  dimension "d37" = 109.8988
  dimension "d38" = 0.9345
  dimension "d39" = 0.9345
  dimension "d40" = 0.9345
  dimension "d41" = 0.9345
  dimension "d50" = 10.769
  dimension "d51" = 12.638
  constraint midpoint L4 L8.start
  constraint midpoint L6 L8.end
  constraint midpoint L7 L9.start
  constraint midpoint L5 L9.end
  constraint horizontal L10
  constraint perpendicular L10 L11
  constraint parallel L10 L12
  constraint parallel L11 L13
  constraint coincident L14 P2
  constraint coincident L15 P2
  constraint midpoint L8 P2
  constraint horizontal L16
  constraint perpendicular L16 L17
  constraint parallel L16 L18
  constraint parallel L17 L19
  constraint coincident L20 P2
  constraint coincident L21 P2
  constraint coincident P2 P1
  constraint horizontal L22
  constraint perpendicular L22 L23
  constraint parallel L22 L27
  constraint parallel L23 L24
  constraint coincident L25 P2
  constraint coincident L26 P2
  constraint coincident L26.start L23
  constraint coincident L26.start L22
  constraint coincident L21.start L17
  constraint coincident L21.start L16
  constraint coincident L25.end L27
  constraint coincident L25.end L23
  constraint tangent A8 L27
  constraint tangent L23 A8
  constraint coincident L20.end L18
  constraint coincident L20.end L17
  constraint tangent L18 A9
  constraint tangent L17 A9
  constraint symmetric L8 A8.start A10.end
  constraint symmetric L8 L23.end L24.start
  constraint symmetric L8 A8 A10
  constraint symmetric L8 L18.start L18.end
  constraint symmetric L8 L17.end L19.start
  constraint symmetric L8 A9 A11
  constraint symmetric L9 A10.end L22.start
  constraint symmetric L9 L24.start L24.end
  constraint symmetric L9 A10 A12
  constraint symmetric L9 L18.end L16.start
  constraint symmetric L9 L19.start L19.end
  constraint symmetric L9 A11 A13
  constraint symmetric L9 A8.start L22.end
  constraint symmetric L9 L23.end L23.start
  constraint symmetric L9 A8 A14
  constraint symmetric L9 L18.start L16.end
  constraint symmetric L9 L17.end L17.start
  constraint symmetric L9 A9 A15
  constraint coincident L23.start A14.start
  constraint coincident L17.start A15.start
  constraint coincident L22.end A14.end
  constraint coincident L16.end A15.end
  measures "d36" distance of L11.end L12.end
  measures "d37" distance of L10.end L11.end
  measures "d38" distance of L13 L19
  measures "d39" distance of L13 L24
  measures "d40" distance of L10 L16
  measures "d41" distance of L10 L22
  measures "d50" radius of A8
  measures "d51" radius of A9
extrude "Extrude6" cut sketch "Sketch5" against normal blind 1.424 contours L16 L17 L18 L19 A9 A11 A13 A15
extrude "Extrude7" cut 1 faces at (17.2514, 2.7546, 0) along direction (0, 0, 1) blind 0.5
sketch "Sketch6" plane through (0, 0, 0.5) normal (0, 0, -1) x (1, 0, 0)
  line L0 (108.2459, 68.2638) -> (-28.2459, 68.2638)
  arc A0 (-28.2459, 68.2638) -> (-38.2638, 58.2459) centre (-28.2459, 58.2459) ccw
  line L1 (-38.2638, 58.2459) -> (-38.2638, -28.2459)
  arc A1 (-38.2638, -28.2459) -> (-28.2459, -38.2638) centre (-28.2459, -28.2459) ccw
  line L2 (-28.2459, -38.2638) -> (108.2459, -38.2638)
  arc A2 (108.2459, -38.2638) -> (118.2638, -28.2459) centre (108.2459, -28.2459) ccw
  line L3 (118.2638, -28.2459) -> (118.2638, 58.2459)
  arc A3 (118.2638, 58.2459) -> (108.2459, 68.2638) centre (108.2459, 58.2459) ccw
  line L4 (40, 68.2638) -> (40, -38.2638) construction
  line L5 (-38.2638, 15) -> (118.2638, 15) construction
  line L6 (96, -27.5) -> (-16, -27.5)
  line L7 (-20, -23.5) -> (-20, 53.5)
  line L8 (-16, 57.5) -> (96, 57.5)
  line L9 (100, 53.5) -> (100, -23.5)
  line L10 (100, -27.5) -> (-20, 57.5) construction
  line L11 (-20, -27.5) -> (100, 57.5) construction
  arc A4 (-16, 57.5) -> (-20, 53.5) centre (-16, 53.5) ccw
  arc A5 (100, 53.5) -> (96, 57.5) centre (96, 53.5) ccw
  arc A6 (96, -27.5) -> (100, -23.5) centre (96, -23.5) ccw
  arc A7 (-20, -23.5) -> (-16, -27.5) centre (-16, -23.5) ccw
  point P0 (40, 15)
  dimension "d58" = 120
  dimension "d59" = 85
  dimension "d68" = 4
  dimension "d69" = 4
  dimension "d70" = 4
  dimension "d71" = 4
  constraint midpoint L0 L4.start
  constraint midpoint L2 L4.end
  constraint midpoint L1 L5.start
  constraint midpoint L3 L5.end
  constraint horizontal L6
  constraint perpendicular L6 L7
  constraint parallel L6 L8
  constraint parallel L7 L9
  constraint coincident L10 P0
  constraint coincident L11 P0
  constraint midpoint L5 P0
  constraint coincident L10.end L8
  constraint coincident L10.end L7
  constraint tangent L8 A4
  constraint tangent L7 A4
  constraint coincident L11.end L8
  constraint coincident L11.end L9
  constraint tangent L8 A5
  constraint tangent L9 A5
  constraint coincident L10.start L9
  constraint coincident L10.start L6
  constraint tangent L9 A6
  constraint tangent L6 A6
  constraint coincident L11.start L7
  constraint coincident L11.start L6
  constraint tangent L7 A7
  constraint tangent L6 A7
  measures "d58" distance of L10.end L11.end
  measures "d59" distance of L11.start L10.end
  measures "d68" radius of A4
  measures "d69" radius of A5
  measures "d70" radius of A6
  measures "d71" radius of A7
extrude "Extrude8" cut sketch "Sketch6" against normal blind 1.1 contours L6 L7 L8 L9 A4 A5 A6 A7